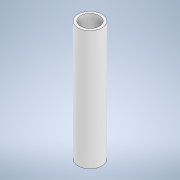
# Autodesk Inventor part: casing
Saved by Autodesk Inventor 2021 (Build 250183000, 183)
## iProperties
Created: 2021-04-18
Part Number: casing
Material: PVC, Unplasticized
Document SubType Name: Modeling
Designer: samlo
Density: 1.29 g/cm^3
Appearance: Smooth - White
Author: samlo
Autodesk Inventor part; units mm, degrees
ref_plane "YZ Plane" through (0, 0, 0) normal (1, 0, 0) x (0, 1, 0)
ref_plane "XZ Plane" through (0, 0, 0) normal (0, 1, 0) x (-1, 0, 0)
ref_plane "XY Plane" through (0, 0, 0) normal (0, 0, 1) x (1, 0, 0)
sketch "Sketch1" plane through (0, 0, 0) normal (0, 0, 1) x (1, 0, 0)
  line L0 (15.5, 0) -> (15.5, 200)
  line L1 (15.5, 200) -> (20, 200)
  line L2 (20, 200) -> (20, 0)
  line L3 (20, 0) -> (15.5, 0)
  line L4 (0, -40) -> (0, 240) projected
  point P0 (0, 0)
  dimension "d1" = 20
  dimension "d2" = 15.5
  dimension "d3" = 200
  constraints: 8 end point, 3 perpendicular, 1 vertical
  measures "d1" distance of L2.end point (0, 0)
  measures "d2" distance of L0.start point (0, 0)
  measures "d3" vertical distance of L0.end point (0, 0)
revolve "Revolution1" add sketch "Sketch1" angle 360 about axis through (0, -10, 0) along (0, 1, 0)
body "Solid1"
